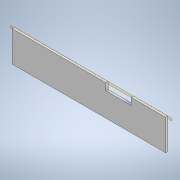
# Autodesk Inventor part: other top
Saved by Autodesk Inventor 2020 (Build 240168000, 168)
## iProperties
Created: 2020-01-17
Part Number: other top
Material: Generic
Document SubType Name: Modeling
Designer: FTC8863
Density: 1 g/cm^3
Appearance: Default
Author: FTC8863
Autodesk Inventor part; units mm, degrees
ref_plane "YZ Plane" through (0, 0, 0) normal (1, 0, 0) x (0, 1, 0)
ref_plane "XZ Plane" through (0, 0, 0) normal (0, 1, 0) x (-1, 0, 0)
ref_plane "XY Plane" through (0, 0, 0) normal (0, 0, 1) x (1, 0, 0)
ref_plane "Work Plane1" through (0, 0, 0) normal (0, 0, 1) x (1, 0, 0)
sketch "Sketch1" plane through (0, 0, 0) normal (0, 0, 1) x (1, 0, 0)
  line L0 (0, 0) -> (450.85, 0) construction
  line L1 (0, -6.35) -> (450.85, -6.35) construction
  line L2 (0, -84.027) -> (450.85, -84.027) construction
  line L3 (0, -90.377) -> (450.85, -90.377) construction
  line L4 (450.85, -90.377) -> (0, -90.377)
  line L5 (0, -90.377) -> (0, 0)
  arc A0 (30.6582, -6.35) -> (0, 0) centre (0, -77.185) ccw
  line L6 (450.85, -90.377) -> (450.85, 0)
  line L7 (349.25, 0) -> (349.25, -20.32)
  line L8 (349.25, -20.32) -> (275.59, -20.32)
  line L9 (275.59, -20.32) -> (275.59, 0)
  line L10 (0, 0) -> (275.59, 0)
  line L11 (349.25, 0) -> (450.85, 0)
  dimension "d2" = 101.6
  dimension "d3" = 73.66
  dimension "d4" = 20.32
  constraints: 16 end point, 3 collinear, 3 perpendicular, 3 tangent, 2 point on circle, 1 centre point, 1 parallel, 1 point on line, 1 vertical
  measures "d2" distance from line of L7 L0.end
  measures "d3" distance between parallel lines of L9 L7
  measures "d4" distance from line of L7.start L8
extrude "Extrusion1" add sketch "Sketch1" along normal blind 6.35
body "Solid1"
